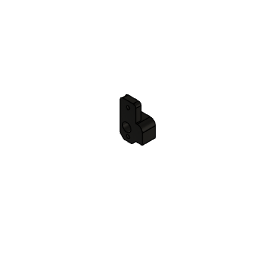
Endstop Buddy (Autodesk Fusion 360 design; units mm, degrees)
Autodesk Fusion 360 part; units mm, degrees
ref_plane "WorkPlane1" through (13, -22, 12.515) normal (0, -1, 0) x (1, 0, 0)
sketch "Sketch1" plane through (21.5, -22, 18.515) normal (0, -1, 0) x (1, 0, 0)
  line L0 (-8.5, -6) -> (8.5, -6)
  line L1 (8.5, -6) -> (8.5, 6)
  line L2 (8.5, 6) -> (-8.5, 6)
  line L3 (-8.5, 6) -> (-8.5, -6)
  line L4 (4.5, 1.85) -> (4.5, -3.85)
  line L5 (4.5, -3.85) -> (1.8, -3.85)
  line L6 (1.8, -3.85) -> (1.8, 1.85)
  line L7 (1.8, 1.85) -> (4.5, 1.85)
extrude "Extrude1" add sketch "Sketch1" along normal blind 10 contours L0 L1 L2 L3 | L4 L5 L6 L7
extrude "Extrude2" add sketch "Sketch1" against normal blind 2 contours L4 L5 L6 L7
move_face "OffsetFaces1" offset -0.1 4 faces at (26, -20.6667, 18.465) (24.2, -21.3333, 20.365) (23.3, -21.3333, 16.565) (25.1, -21.3333, 14.665)
chamfer "Chamfer1" distance 0.5 angle 45 4 edges at (25.9, -21, 20.265) (23.4, -21, 20.265) (23.4, -21, 14.765) (25.9, -21, 14.765)
sketch "Sketch2" plane through (0, -32, 0) normal (0, -1, 0) x (1, 0, 0)
  line L0 (13, 24.515) -> (13, 12.515)
  line L1 (13, 12.515) -> (30, 12.515)
  line L2 (30, 12.515) -> (30, 24.515)
  line L3 (30, 24.515) -> (13, 24.515)
  line L4 (13, 36.515) -> (25, 36.515)
  line L5 (25, 36.515) -> (25, 9.515)
  line L6 (25, 9.515) -> (13, 9.515)
  line L7 (13, 9.515) -> (13, 36.515)
  dimension "d7187" = 12
  dimension "d7188" = 27
  dimension "d7189" = 3
  dimension "d7190" = 12
  constraint horizontal L4
  constraint vertical L5
  constraint horizontal L6
  constraint vertical L7
  constraint coincident L0.start L7
  measures "d7187" distance of L4.start L4.end
  measures "d7188" distance of L4.start L6.end
  measures "d7189" distance of L1 L6
  measures "d7190" distance of L3 L4
extrude "Extrude3" add sketch "Sketch2" against normal blind 2 contours L3 L4 L5 L7 | L1 L5 L6 L7
extrude "Extrude4" add 1 faces at (21, -30, 28.515) along direction (0, 1, 0) blind 2
sketch "Sketch3" plane through (0, -32, 0) normal (0, -1, 0) x (1, 0, 0)
  line L0 (13, 36.515) -> (13, 9.515)
  line L1 (13, 9.515) -> (25, 9.515)
  line L2 (25, 9.515) -> (25, 12.515)
  line L3 (25, 12.515) -> (30, 12.515)
  line L4 (30, 12.515) -> (30, 24.515)
  line L5 (30, 24.515) -> (25, 24.515)
  line L6 (25, 24.515) -> (25, 36.515)
  line L7 (25, 36.515) -> (13, 36.515)
  line L8 (13, 32.015) -> (19, 32.015)
  line L9 (19, 32.015) -> (19, 12.765)
  dimension "d7195" = 90
  dimension "d7196" = 19.25
  dimension "d7197" = 6
  dimension "d7198" = 4.5
  constraint coincident L0 L8.start
  constraint perpendicular L0 L8
  measures "d7195" angle of L8 L9
  measures "d7196" distance of L8.end L9.end
  measures "d7197" distance of L8.start L8.end
  measures "d7198" distance of L7 L8
hole "Hole1" at (19, -32, 32.015) at (19, -32, 12.765) direction (0, 1, 0) diameter 2.5 depth 10 tip angle 180
chamfer "Chamfer2" distance 3 angle 45 2 edges at (25, -31, 9.515) (13, -31, 9.515)
fillet "Fillet1" radius 2 2 edges at (25, -30, 36.515) (13, -30, 36.515)
fillet "Fillet1" radius 4 2 edges at (30, -27, 24.515) (13, -25, 24.515)
sketch "Sketch4" plane through (0, -32, 0) normal (0, -1, 0) x (1, 0, 0)
  arc A0 (30, 20.515) -> (26, 24.515) centre (26, 20.515) ccw
  line L0 (26, 24.515) -> (25, 24.515)
  line L1 (25, 24.515) -> (25, 34.515)
  arc A1 (25, 34.515) -> (23, 36.515) centre (23, 34.515) ccw
  line L2 (23, 36.515) -> (15, 36.515)
  arc A2 (15, 36.515) -> (13, 34.515) centre (15, 34.515) ccw
  line L3 (13, 34.515) -> (13, 12.515)
  line L4 (13, 12.515) -> (16, 9.515)
  line L5 (16, 9.515) -> (22, 9.515)
  line L6 (22, 9.515) -> (25, 12.515)
  line L7 (25, 12.515) -> (30, 12.515)
  line L8 (30, 12.515) -> (30, 20.515)
  circle A3 centre (19, 32.015) radius 1.25
  circle A4 centre (19, 12.765) radius 1.25
  circle A5 centre (18, 18.515) radius 1.25
hole "Hole2" at (18, -32, 18.515) direction (0, 1, 0) diameter 2.5 depth 16 tip angle 180 counterbore diameter 6.5 counterbore depth 5
move_face "OffsetFaces2" offset -0.25 1 faces at (18.0623, -25.3333, 17.2666)
sketch "Sketch5" plane through (0, -27, 0) normal (0, -1, 0) x (1, 0, 0)
  circle A0 centre (18, 18.515) radius 3.25
  circle A1 centre (18, 18.515) radius 1.5
extrude "Extrude5" add sketch "Sketch5" against normal blind 0.25 contours A1
